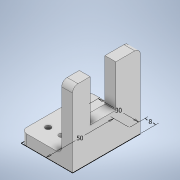
# Autodesk Inventor part: Part1
Saved by Autodesk Inventor 2020.3 (Build 243373000, 373)
## iProperties
Created: 2020-07-15
Part Number: Part1
Material: Generic
Document SubType Name: Modeling
Designer: mifer
Density: 1 g/cm^3
Appearance: Default
Author: mifer
## iProperties of the stored document _3DPrint.ipt
Created: 2020-08-25
Part Number: _3DPrint
Material: Generic
Document SubType Name: Modeling
Designer: mifer
Density: 1 g/cm^3
Appearance: Default
Author: mifer
Autodesk Inventor part; units mm, degrees
ref_plane "YZ Plane" through (0, 0, 0) normal (1, 0, 0) x (0, 1, 0)
ref_plane "XZ Plane" through (0, 0, 0) normal (0, 1, 0) x (-1, 0, 0)
ref_plane "XY Plane" through (0, 0, 0) normal (0, 0, 1) x (1, 0, 0)
sketch "Sketch1" plane through (0, 0, 0) normal (0, 1, 0) x (-1, 0, 0)
  line L0 (0, 0) -> (8, 0)
  line L1 (8, 0) -> (8, -50)
  line L2 (8, -50) -> (0, -50)
  line L3 (0, -50) -> (0, 0)
  line L4 (8, 0) -> (38, 0)
  line L5 (38, 0) -> (38, -50)
  line L6 (38, -50) -> (8, -50)
  line L7 (8, -50) -> (8, 0)
  circle A0 centre (30, -12) radius 2
  circle A1 centre (20, -12) radius 2
  circle A2 centre (30, -25) radius 2
  circle A3 centre (20, -25) radius 2
  circle A4 centre (30, -38) radius 2
  circle A5 centre (20, -38) radius 2
  dimension "d15" = 8
  dimension "d16" = 50
  dimension "d17" = 30
  constraints: 16 end point, 6 centre point, 4 parallel, 2 horizontal, 2 perpendicular
  measures "d15" distance of L1.end L2.end
  measures "d16" distance of L0.end L1.end
  measures "d17" distance of L5.end L6.end
extrude "Extrusion3" add sketch "Sketch1" along normal blind 8 contours L4 L5 L6 L1
extrude "Extrusion4" add sketch "Sketch1" along normal blind 55 contours L0 L1 L2 L3
fillet "Fillet1" radius 4 1 edges at (-8, 8, -25)
sketch "Sketch2" plane through (0, 0, 0) normal (1, 0, 0) x (0, 0, -1)
  line L0 (50, 0) -> (0, 0) projected
  line L1 (10, 8) -> (10, 0) projected
  circle A0 centre (7, 36) radius 2
  circle A1 centre (42, 36) radius 2
  line L2 (50, 0) -> (50, 55) projected
  line L3 (37, 36) -> (37, 24)
  line L4 (37, 24) -> (18, 24)
  line L5 (18, 24) -> (18, 55)
  line L6 (37, 36) -> (37, 55)
  line L7 (18, 55) -> (37, 55)
  line L8 (13, 55) -> (13, 48)
  line L9 (13, 55) -> (32, 55)
  line L10 (32, 55) -> (32, 24)
  line L11 (32, 24) -> (13, 24)
  line L12 (13, 24) -> (13, 55)
  point P0 (0, 55)
  dimension "d31" = 50
  dimension "d32" = 35
  dimension "d33" = 8
  dimension "d34" = 13
  dimension "d36" = 19
  constraints: 20 end point, 3 parallel, 3 perpendicular, 2 centre point, 1 horizontal, 1 point on line
  measures "d31" distance of L0.start L0.end
  measures "d32" distance of A1.centre A0.centre
  measures "d33" distance from line of L2 A1.centre
  measures "d34" distance between parallel lines of L2 L6
  measures "d36" distance between parallel lines of L6 L5
fillet "Fillet2" radius 4 4 edges at (-4, 55, -50) (-4, 55, 0) (-38, 4, 0) (-38, 4, -50)
extrude "Extrusion6" cut sketch "Sketch2" against normal blind 10 contours L4 L5 L7 L10 | L11 L12 L8 L9 L5
body "Solid2"
